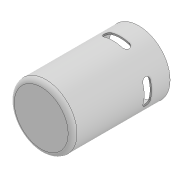
# Autodesk Inventor part: motor
Saved by Autodesk Inventor 2020 (Build 240168000, 168)
## iProperties
Created: 2020-08-28
Part Number: motor
Material: 일반
Document SubType Name: Modeling
Designer: 이호석
Mass: 9.3559 g
Surface Area: 190.191 cm^2
Volume: 9.3559 cm^3
Density: 1 g/cm^3
Appearance: 기본값
Author: 이호석
Autodesk Inventor part; units mm, degrees
ref_plane "YZ Plane" through (0, 0, 0) normal (1, 0, 0) x (0, 1, 0)
ref_plane "XZ Plane" through (0, 0, 0) normal (0, 1, 0) x (-1, 0, 0)
ref_plane "XY Plane" through (0, 0, 0) normal (0, 0, 1) x (1, 0, 0)
sketch "스케치1" plane through (0, 0, 0) normal (0, 0, 1) x (1, 0, 0)
  circle A0 centre (0, 0) radius 21.2
  dimension "d0" = 42.4
  constraints: 1 centre point, 1 coincident
  measures "d0" diameter of A0
extrude "돌출1" add sketch "스케치1" along normal blind 30
sketch "스케치2" plane through (0, 0, 30) normal (0, 0, 1) x (1, 0, 0)
  circle A0 centre (0, 0) radius 21.2
  dimension "d3" = 42.4
  constraints: 1 centre point, 1 coincident
  measures "d3" diameter of A0
extrude "돌출2" add sketch "스케치2" along normal blind 30
sketch "스케치3" plane through (0, 0, 60) normal (0, 0, 1) x (1, 0, 0)
  circle A0 centre (0, 0) radius 21.2
  dimension "d6" = 42.4
  constraints: 1 centre point, 1 coincident
  measures "d6" diameter of A0
extrude "돌출3" add sketch "스케치3" along normal blind 6
fillet "모깎기1" radius 3 1 edges at (-21.2, 0, 66)
shell "쉘1" thickness 1 removed faces 1 at (2.7392, 4.6861, 0)
ref_plane "작업 평면1" through (0, 21.2, 0) normal (0, 1, 0) x (-1, 0, 0)
sketch "스케치12" plane through (0, 21.2, 0) normal (0, 1, 0) x (-1, 0, 0)
  line L0 (0, 0) -> (0, 60)
  line L1 (0, 60) -> (0, 30)
  line L2 (0, 30) -> (0, 15)
  line L3 (-6, 15) -> (6, 15) construction
  line L4 (-6, 12.5) -> (6, 12.5)
  line L5 (6, 17.5) -> (-6, 17.5)
  arc A0 (-6, 17.5) -> (-6, 12.5) centre (-6, 15) ccw
  arc A1 (6, 12.5) -> (6, 17.5) centre (6, 15) ccw
  dimension "d47" = 60
  dimension "d48" = 30
  dimension "d49" = 15
  dimension "d50" = 6
  dimension "d51" = 5
  constraints: 14 end point, 4 point on circle, 4 tangent, 2 centre point, 2 midpoint, 1 parallel, 1 perpendicular, 1 point on line, 1 vertical
  measures "d47" distance of L0.start L0.end
  measures "d48" distance of L0.end L1.end
  measures "d49" distance of L1.end L2.end
  measures "d50" distance of L2.end L3.end
  measures "d51" diameter of A1
extrude "돌출12" cut sketch "스케치12" against normal through all
pattern_circular "원형 패턴2" count 4 over 360 about axis through (0, 0, 0) along (0, 0, 1) of "돌출12"
sketch "스케치13" plane through (0, 0, 0) normal (0, 0, -1) x (-1, 0, 0)
  line L0 (0, 0) -> (0, -4)
  line L1 (0, -4) -> (0, 4)
  line L2 (0, 4) -> (20.8192, 4)
  circle A0 centre (0, 0) radius 21.2 projected
  line L3 (0, -4) -> (20.8192, -4)
  dimension "d61" = 4
  dimension "d62" = 8
  constraints: 8 end point, 2 point on circle, 1 parallel, 1 perpendicular, 1 point on line, 1 vertical
  measures "d61" distance of L0.start L0.end
  measures "d62" distance of L0.end L1.end
extrude "돌출13" cut sketch "스케치13" against normal blind 5 contours L1 L2 A0 L3 L0 picked at (6.9397, -2.6667)
